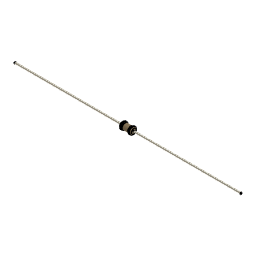
Resistor v1 (Autodesk Fusion 360 design; units mm, degrees)
Autodesk Fusion 360 part; units mm, degrees
note: some values were not read from the file. Set by a fixed rule: which sketch regions a step uses.
sketch "Sketch1" plane through (0, 0, 0) normal (1, 0, 0) x (0, 1, 0) in component "Resistor"
  circle A0 centre (0, 0) radius 0.9
  dimension "d1" = 1.8
  constraint coincident A0.centre origin
  measures "d1" diameter of A0
extrude "Extrude1" add sketch "Sketch1" along normal blind 3 makes body 1 in component "Resistor"
sketch "Sketch2" plane through (3, 0, 0) normal (1, 0, 0) x (0, 1, 0) in component "Resistor"
  circle A0 centre (0, 0) radius 0.9
  circle A1 centre (0, 0) radius 0.225
  dimension "d4" = 0.45
  constraint concentric A0 A1
  measures "d4" diameter of A1
extrude "Extrude2" add sketch "Sketch2" along normal blind 28 separate body contours A1 makes body 2 in component "Resistor"
sketch "Sketch3" plane through (0, 0, 0) normal (-1, 0, 0) x (0, -1, 0) in component "Resistor"
  circle A0 centre (0, 0) radius 0.9
  circle A1 centre (0, 0) radius 0.225
  dimension "d7" = 0.45
  constraint concentric A0 A1
  measures "d7" diameter of A1
extrude "Extrude3" add sketch "Sketch3" along normal blind 28 separate body contours A1 makes body 3 in component "Resistor"
fillet "Fillet1" radius 0.25 2 edges at (3, -0.8391, -0.3255) (0, -0.8391, -0.3255) on bodies 1 in component "Resistor"
sketch "Sketch4" plane through (0, 0, 0) normal (0, 1, 0) x (1, 0, 0) in component "Resistor"
  spline S0 degree 5 poles (0.5, -0.9) (0.58, -0.9) (0.74, -0.9) (0.98, -0.9) (1.3, -0.9) (1.7, -0.9) (2.02, -0.9) (2.26, -0.9) (2.42, -0.9) (2.5, -0.9) knots 0 0 0 0 0 0 0.2 0.4 0.6 0.8 1 1 1 1 1 1
  line L0 (0.5, -0.9) -> (2.5, -0.9)
  line L1 (0.5, -0.9) -> (0.75, -0.7981)
  line L2 (0.75, -0.7981) -> (2.25, -0.7981)
  line L3 (2.25, -0.7981) -> (2.5, -0.9)
  dimension "d14" = 0.25
  dimension "d15" = 1.5
  dimension "d16" = 0.25
  constraint horizontal L0
  constraint parallel L0 L2
  measures "d14" distance of S0.start L1.end
  measures "d15" distance of L1.end L2.end
  measures "d16" distance of S0.end L2.end
revolve "Revolve1" cut sketch "Sketch4" angle 360 about axis through (0, 0, 0) along (-1, 0, 0) bodies 1 in component "Resistor"
sketch "Sketch5" plane through (0, 0, 0) normal (0, 1, 0) x (1, 0, 0) in component "Resistor"
component "Resistor" placed x (1, 0, 0) y (0, 1, 0) z (0, 0, 1) at (0, 0, 0)
equation "d15 = d14 * 6"
equation "d16 = d14"
